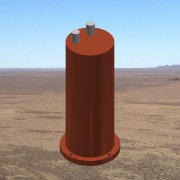
# Autodesk Inventor part: balun
Saved by Autodesk Inventor 2014 SP1 (Build 180222100, 222)
## iProperties
Created: 2014-07-14
Part Number: balun
Material: Copper
Document SubType Name: Modeling
Designer: Dave
Density: 8.94 g/cm^3
Appearance: Copper - Satin
Mass: 306.415 g
Surface Area: 500.792 cm^2
Volume: 34.2746 cm^3
Author: Dave
Autodesk Inventor part; units mm, degrees
ref_plane "YZ Plane" through (0, 0, 0) normal (1, 0, 0) x (0, 1, 0)
ref_plane "XZ Plane" through (0, 0, 0) normal (0, 1, 0) x (-1, 0, 0)
ref_plane "XY Plane" through (0, 0, 0) normal (0, 0, 1) x (1, 0, 0)
sketch "Sketch1" plane through (0, 0, 0) normal (0, 1, 0) x (-1, 0, 0)
  circle A0 centre (0, 0) radius 31.75
  circle A1 centre (0, 0) radius 25.527
  dimension "d0" = 63.5
  dimension "d1" = 6.223
  constraints: 2 centre point, 1 coincident
  measures "d0" diameter of A0
  measures "d1" radial gap between concentric circles of A1 A0
extrude "Extrusion1" add sketch "Sketch1" along normal blind 6.35
sketch "Sketch2" plane through (0, 6.35, 0) normal (0, 1, 0) x (1, 0, 0)
  circle A0 centre (0, 0) radius 25.527 projected
  circle A1 centre (0, 28.575) radius 1.535
  dimension "d4" = 28.575
  constraints: 1 centre point
  measures "d4" distance of A1.centre A0.centre
hole "Hole1" at (0, 6.35, -28.575) direction (0, -1, 0) diameter 3.3528 depth 25.4 tip angle 118
pattern_circular "Circular Pattern1" count 4 over 360 about axis through (0, 0, 0) along (0, 1, 0) of "Hole1"
sketch "Sketch4" plane through (0, 0, 0) normal (0, -1, 0) x (1, 0, 0)
  circle A0 centre (0, 0) radius 25.527 projected
  circle A1 centre (0, 0) radius 24.765
  dimension "d16" = 0.762
  constraints: 1 centre point
  measures "d16" radial gap between concentric circles of A1 A0
extrude "Extrusion2" add sketch "Sketch4" against normal blind 137.16
sketch "Sketch5" plane through (0, 137.16, 0) normal (0, 1, 0) x (1, 0, 0)
  circle A0 centre (0, 0) radius 24.765 projected
extrude "Extrusion3" add sketch "Sketch5" against normal blind 4.826
sketch "Sketch6" plane through (0, 137.16, 0) normal (0, 1, 0) x (1, 0, 0)
  circle A0 centre (0, 0) radius 25.527 projected
  circle A1 centre (-10.414, 10.922) radius 4.445
  line L0 (0, 0) -> (-12.3032, 0) construction
  circle A2 centre (-10.414, -10.922) radius 4.445
  dimension "d21" = 10.414
  dimension "d22" = 10.922
  dimension "d23" = 8.89
  constraints: 2 centre point, 2 end point, 1 horizontal, 1 symmetric about line, 1 other
  measures "d21" horizontal distance of A1.centre L0.start
  measures "d22" vertical distance of A1.centre L0.start
  measures "d23" diameter of A1
extrude "Extrusion4" add sketch "Sketch6" along normal blind 12.7 contours A1 | A2
body "Solid1"
